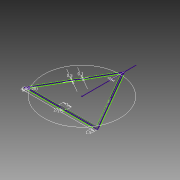
# Autodesk Inventor part: Triangle
Saved by Autodesk Inventor 2015 (Build 190159000, 159)
## iProperties
Created: 2016-08-08
Part Number: Triangle
Material: Generic
Document SubType Name: Modeling
Designer: Javier
Density: 1 g/cm^3
Appearance: Default
Author: Javier
Autodesk Inventor part; units mm, degrees
ref_plane "YZ Plane" through (0, 0, 0) normal (1, 0, 0) x (0, 1, 0)
ref_plane "XZ Plane" through (0, 0, 0) normal (0, 1, 0) x (-1, 0, 0)
ref_plane "XY Plane" through (0, 0, 0) normal (0, 0, 1) x (1, 0, 0)
sketch "Sketch2" plane through (0, 0, 0) normal (0, 1, 0) x (-1, 0, 0)
  line L0 (0, -158.194) -> (-137, 79.097)
  line L1 (-137, 79.097) -> (137, 79.097)
  line L2 (137, 79.097) -> (0, -158.194)
  line L3 (0, -156.194) -> (-135.2679, 78.097)
  line L4 (-135.2679, 78.097) -> (135.2679, 78.097)
  line L5 (135.2679, 78.097) -> (0, -156.194)
  line L6 (0, -148.194) -> (-128.3397, 74.097)
  line L7 (-128.3397, 74.097) -> (128.3397, 74.097)
  line L8 (128.3397, 74.097) -> (0, -148.194)
  line L9 (0, 0) -> (0, -202.1847)
  line L10 (122, 72.7976) -> (-122, 72.7976)
  line L11 (-122, 72.7976) -> (-122, 81.133)
  line L12 (-122, 81.133) -> (122, 81.133)
  line L13 (122, 81.133) -> (122, 72.7976)
  line L14 (0, 72.7976) -> (0, 81.133)
  line L15 (-15, 72.7976) -> (-15, 81.133)
  line L16 (15, 72.7976) -> (15, 81.133)
  line L17 (-124.0446, 69.2563) -> (-2.0446, -142.0539)
  line L18 (-2.0446, -142.0539) -> (-9.2633, -146.2216)
  line L19 (-9.2633, -146.2216) -> (-131.2633, 65.0886)
  line L20 (-131.2633, 65.0886) -> (-124.0446, 69.2563)
  line L21 (-63.0446, -36.3988) -> (-70.2633, -40.5665)
  line L22 (-55.5446, -49.3892) -> (-62.7633, -53.5569)
  line L23 (-70.5446, -23.4084) -> (-77.7633, -27.5761)
  line L24 (2.0446, -142.0539) -> (124.0446, 69.2563)
  line L25 (124.0446, 69.2563) -> (131.2633, 65.0886)
  line L26 (131.2633, 65.0886) -> (9.2633, -146.2216)
  line L27 (9.2633, -146.2216) -> (2.0446, -142.0539)
  line L28 (63.0446, -36.3988) -> (70.2633, -40.5665)
  line L29 (70.5446, -23.4084) -> (77.7633, -27.5761)
  line L30 (55.5446, -49.3892) -> (62.7633, -53.5569)
  dimension "d34" = 1
  dimension "d35" = 5
  dimension "d36" = 274
  dimension "d37" = 0
  dimension "d51" = 15
  dimension "d52" = 15
  dimension "d53" = 15
  dimension "d54" = 30
  dimension "d57" = 360
  constraints: 62 end point, 12 point on line, 3 coincident, 3 perpendicular, 2 midpoint, 2 parallel, 1 horizontal, 1 vertical, 73 other
  measures "d34" distance between parallel lines of L2 L5
  measures "d35" distance between parallel lines of L2 L8
  measures "d36" distance of L0.end L1.end
  measures "d37" distance from line of L9 L0.start
  measures "d51" horizontal distance of L11.end L0.end
  measures "d52" distance from line of L1.end L13
  measures "d53" distance between parallel lines of L15 L14
  measures "d54" distance between parallel lines of L16 L15
extrude "Extrusion7" add sketch "Sketch2" along normal blind 10 contours L9 L5 L27 L2 | L0 L18 L3 L9 | L0 L22 L3 L18 | L27 L5 L30 L2 | L0 L21 L3 L22 | L30 L5 L28 L2 | L0 L23 L3 L21 | L28 L5 L29 L2 | L0 L20 L3 L23 | L29 L5 L25 L2 | L0 L1 L11 L4 L3 L20 | L25 L5 L4 L13 L1 L2 | L1 L15 L4 L11 | L13 L4 L16 L1 | L1 L14 L4 L15 | L16 L4 L14 L1
extrude "Extrusion8" add sketch "Sketch2" along normal blind 1 contours L9 L8 L27 L5 | L3 L18 L6 L9 | L3 L22 L6 L18 | L27 L8 L30 L5 | L3 L21 L6 L22 | L30 L8 L28 L5 | L3 L23 L6 L21 | L28 L8 L29 L5 | L3 L20 L6 L23 | L29 L8 L25 L5 | L3 L4 L11 L7 L6 L20 | L25 L8 L7 L13 L4 L5 | L4 L15 L7 L11 | L13 L7 L16 L4 | L4 L14 L7 L15 | L16 L7 L14 L4
fillet "Fillet3" radius 1 3 edges at (-67.634, 1, -39.0485) (67.634, 1, -39.0485) (0, 1, 78.097)
extrude "Extrusion10" cut sketch "Sketch2" along normal blind 7.5 contours L18 L19 L22 L0 | L0 L22 L3 L18 | L27 L5 L30 L2 | L2 L30 L26 L27 | L3 L22 L6 L18 | L27 L8 L30 L5 | L6 L22 L17 L18 | L27 L24 L30 L8 | L23 L19 L20 L0 | L0 L20 L3 L23 | L29 L5 L25 L2 | L2 L25 L26 L29 | L3 L20 L6 L23 | L29 L8 L25 L5 | L6 L20 L17 L23 | L29 L24 L25 L8 | L11 L12 L15 L1 | L1 L15 L4 L11 | L13 L4 L16 L1 | L1 L16 L12 L13 | L4 L15 L7 L11 | L13 L7 L16 L4 | L7 L15 L10 L11 | L13 L10 L16 L7
sketch "Sketch3" plane through (0, 0, 0) normal (0, -1, 0) x (1, 0, 0)
  line L0 (177.2057, 67.9092) -> (177.2057, 204.1642)
  line L1 (177.2057, 204.1642) -> (0, 204.1642)
  line L2 (0, 204.1642) -> (0, 67.9092)
  line L3 (61, -52.5389) -> (76, -26.5581) projected
  line L4 (68.5, -39.5485) -> (60.9094, -35.1661)
  line L5 (60.9094, -35.1661) -> (0, 67.9092)
  line L6 (68.5, -39.5485) -> (177.2057, 67.9092)
  point P0 (0, 0)
  constraints: 12 end point, 1 midpoint, 1 parallel, 1 perpendicular
extrude "Extrusion11" cut sketch "Sketch3" against normal blind 1000 keep common part
sketch "Sketch4" plane through (0, 0, 74.097) normal (-1, 0, 0) x (0, 0, 1)
  line L0 (5, 0) -> (0, 0)
  line L1 (0, 0) -> (0, 7.5)
  line L2 (0, 7.5) -> (5, 7.5)
  line L3 (5, 7.5) -> (5, 0)
  point P0 (-74.097, 0)
  constraints: 8 end point, 2 parallel, 1 horizontal, 1 perpendicular
extrude "Extrusion12" add sketch "Sketch4" against normal blind 1
sketch "Sketch5" plane through (68.5, 0, -39.5485) normal (-0.5, 0, -0.866) x (-0.866, 0, 0.5)
  line L0 (0, 0) -> (5, 0)
  line L1 (5, 0) -> (5, 7.5)
  line L2 (5, 7.5) -> (0, 7.5)
  line L3 (0, 7.5) -> (0, 0)
  point P0 (79.097, 0)
  constraints: 8 end point, 2 parallel, 1 horizontal, 1 perpendicular
extrude "Extrusion13" add sketch "Sketch5" against normal blind 1
body "Solid3"
